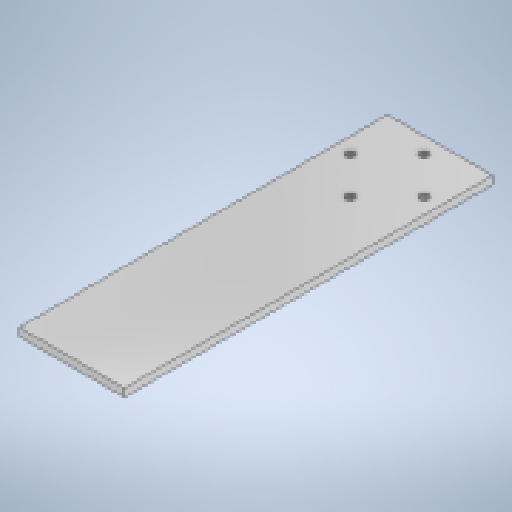
# Autodesk Inventor part: axis_8_10_connector_frame
Saved by Autodesk Inventor 2025.2 (Build 292293000, 293)
## iProperties
Created: 2025-05-04
Part Number: axis_8_10_connector_frame
Material: Aluminum 6061-AHC
Document SubType Name: Sheet Metal
Designer: User
Density: 2.7 g/cm^3
Sheet Metal Rule: Default_mm
Appearance: Aluminum - Dark
Author: User
Autodesk Inventor part; units mm, degrees
ref_plane "YZ Plane" through (0, 0, 0) normal (1, 0, 0) x (0, 1, 0)
ref_plane "XZ Plane" through (0, 0, 0) normal (0, 1, 0) x (-1, 0, 0)
ref_plane "XY Plane" through (0, 0, 0) normal (0, 0, 1) x (1, 0, 0)
sketch "Sketch1" plane through (0, 0, 0) normal (0, 1, 0) x (-1, 0, 0)
  line L0 (10, -35) -> (-10, -35)
  line L1 (-10, -35) -> (-10, 35)
  line L2 (-10, 35) -> (10, 35)
  line L3 (10, 35) -> (10, -35)
  point P0 (0, 0)
  dimension "d0" = 20
  dimension "d1" = 70
  dimension "d2" = 35
  dimension "d3" = 10
  measures "d0" distance of L0.start L0.end
  measures "d1" distance of L0.end L1.end
  measures "d2" distance from line of L0 point (0, 0)
  measures "d3" distance from line of point (0, 0) L1
extrude "Plate1" add sketch "Sketch1" along normal blind 1.5
sketch "Sketch2" plane through (0, 1.5, 0) normal (0, 1, 0) x (1, 0, 0)
  circle A0 centre (-7, 24.9) radius 0.7835 projected
  circle A1 centre (0, 31.9) radius 0.7835 projected
  circle A2 centre (7, 24.9) radius 0.7835 projected
  circle A3 centre (0, 17.9) radius 0.7835 projected
  point P0 (0, 0)
hole "Hole1" at (0, 1.5, -31.9) at (-7, 1.5, -24.9) at (0, 1.5, -17.9) at (7, 1.5, -24.9) direction (0, -1, 0) diameter 1.6 depth 1.5
equation "\"d10\" = Thickness"
equation "\"d4\" = Thickness"
equation "\"BendReliefWidth\" = Thickness"
equation "\"BendReliefDepth\" = 0.5 * Thickness"
equation "\"CornerReliefSize\" = 4 * Thickness"
equation "\"MinimumRemnant\" = 2 * Thickness"
equation "\"TransitionRadius\" = BendRadius"
equation "\"JacobiRadiusSize\" = BendRadius"
equation "\"GapSize\" = Thickness"
equation "\"Thickness\" = 1.5"
equation "\"BendRadius\" = 0.31"
body "Solid1"
